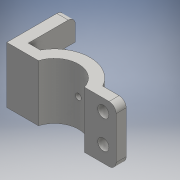
# Autodesk Inventor part: 240628_final3
Saved by Autodesk Inventor 2016 (Build 200138000, 138)
## iProperties
Created: 2024-06-28
Part Number: 240628_final3
Material: 일반
Document SubType Name: Modeling
Designer: pc
Density: 1 g/cm^3
Appearance: 기본값
Author: pc
Autodesk Inventor part; units mm, degrees
ref_plane "YZ Plane" through (0, 0, 0) normal (1, 0, 0) x (0, 1, 0)
ref_plane "XZ Plane" through (0, 0, 0) normal (0, 1, 0) x (-1, 0, 0)
ref_plane "XY Plane" through (0, 0, 0) normal (0, 0, 1) x (1, 0, 0)
sketch "스케치1" plane through (0, 0, 0) normal (0, 0, 1) x (1, 0, 0)
  line L0 (38.7711, -20.2424) -> (-38.7711, -20.2424)
  line L1 (-38.7711, -20.2424) -> (-38.7711, 20.2424)
  line L2 (-38.7711, 20.2424) -> (38.7711, 20.2424)
  line L3 (38.7711, 20.2424) -> (38.7711, -20.2424)
  line L4 (38.7711, -20.2424) -> (-38.7711, 20.2424) construction
  line L5 (-38.7711, -20.2424) -> (38.7711, 20.2424) construction
  point P0 (0, 0)
  constraints: 12 end point, 2 midpoint, 2 parallel, 1 horizontal, 1 perpendicular
extrude "돌출1" add sketch "스케치1" along normal blind 40
sketch "스케치2" plane through (0, 0, 40) normal (0, 0, 1) x (1, 0, 0)
  line L0 (38.7711, 20.2424) -> (-38.7711, 20.2424) projected
  line L1 (-30.6833, 20.2424) -> (-30.6833, -13.1037)
  line L2 (-30.6833, -13.1037) -> (-22.1205, -13.1037)
  line L3 (38.7711, -20.2424) -> (38.7711, 20.2424) projected
  line L4 (38.7711, -13.1037) -> (22.0956, -13.1037)
  arc A0 (22.0956, -13.1037) -> (-22.1205, -13.1037) centre (-0.0125, -25.2018) ccw
  line L5 (-30.6833, 20.2424) -> (38.7711, 20.2424)
  line L6 (38.7711, -13.1037) -> (38.7711, 20.2424)
  circle A1 centre (-0.0125, -25.2018) radius 17.0581
  point P0 (0, 0)
  constraints: 10 end point, 3 point on circle, 2 centre point, 2 horizontal, 2 perpendicular, 2 point on line, 1 coincident, 1 vertical
extrude "돌출2" cut sketch "스케치2" against normal blind 40
sketch "스케치3" plane through (-38.7711, -20.2424, 0) normal (0, -1, 0) x (1, 0, 0)
  circle A0 centre (38.7711, 19.9954) radius 2.1048
  point P0 (38.7711, 0)
  constraints: 1 centre point
extrude "돌출3" cut sketch "스케치3" against normal blind 30.75
sketch "스케치4" plane through (22.0956, -13.1037, 40) normal (0, 1, 0) x (1, 0, 0)
  circle A0 centre (7.6344, 28.4237) radius 4
  circle A1 centre (7.6344, 8.2529) radius 4
  point P0 (-22.0956, 40)
  dimension "d7" = 8
  dimension "d8" = 8
  constraints: 2 centre point
  measures "d7" diameter of A0
  measures "d8" diameter of A1
extrude "돌출4" cut sketch "스케치4" against normal blind 30.75
sketch "스케치5" plane through (-30.6833, -13.1037, 40) normal (1, 0, 0) x (0, 0, -1)
  line L0 (16, 33.3461) -> (16, 22.7148)
  line L1 (0, 33.3461) -> (40, 33.3461) projected
  line L2 (24, 33.3461) -> (24, 19.5161)
  line L3 (40, 33.3461) -> (40, 0) projected
  line L4 (0, 0) -> (0, 33.3461) projected
  arc A0 (16, 19.5161) -> (24, 19.5161) centre (20, 19.5161) ccw
  line L5 (16, 33.3461) -> (24, 33.3461)
  line L6 (16, 19.5161) -> (16, 22.7148)
  point P0 (40, 13.1037)
  dimension "d11" = 16
  dimension "d12" = 16
  constraints: 8 end point, 3 vertical, 2 point on circle, 2 point on line, 2 tangent, 1 centre point, 1 horizontal
  measures "d11" distance between parallel lines of L3 L2
  measures "d12" distance between parallel lines of L4 L0
extrude "돌출5" cut sketch "스케치5" against normal blind 30.75
fillet "모깎기1" radius 5 4 edges at (-34.7272, 20.2424, 40) (-34.7272, 20.2424, 0) (38.7711, -16.673, 40) (38.7711, -16.673, 0)
